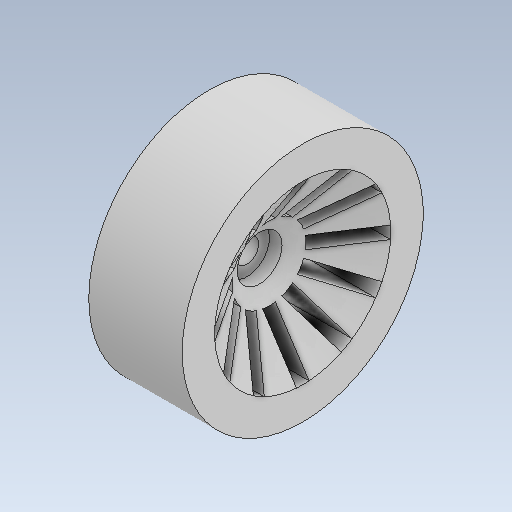
# Autodesk Inventor part: 04_Wheel
Saved by Autodesk Inventor 2021 (Build 250183000, 183)
## iProperties
Created: 2021-03-22
Part Number: 04_Wheel
Material: Generisch
Document SubType Name: Modeling
Designer: User
Density: 1 g/cm^3
Appearance: Vorgabe
Author: User
Autodesk Inventor part; units mm, degrees
ref_plane "YZ Plane" through (0, 0, 0) normal (1, 0, 0) x (0, 1, 0)
ref_plane "XZ Plane" through (0, 0, 0) normal (0, 1, 0) x (-1, 0, 0)
ref_plane "XY Plane" through (0, 0, 0) normal (0, 0, 1) x (1, 0, 0)
derived "00_Mastersketch.ipt"
sketch "05_wheelSketch" plane through (67, -17.95, 0) normal (0, 1, 0) x (-1, 0, 0)
  line L0 (-30, 33.5) -> (-4, 33.5) construction
  line L1 (-4, 33.5) -> (-4, -33.5) construction
  line L2 (-4, -33.5) -> (-30, -33.5) construction
  line L3 (-30, -33.5) -> (-30, 33.5) construction
  line L4 (-18, 16) -> (-30, 33.5) construction
  line L5 (-18, -16) -> (-18, 16) construction
  line L6 (-30, -33.5) -> (-18, -16) construction
  line L7 (-18, -6.25) -> (-4, -6.25) construction
  line L8 (-18, 6.25) -> (-4, 6.25) construction
  line L9 (-4, 0) -> (-30, 0)
  line L10 (-4, 33.5) -> (-30, 33.5)
  line L11 (-4, 33.5) -> (-4, 24.5)
  line L12 (-4, 24.5) -> (-30, 24.5)
  line L13 (-30, 24.5) -> (-30, 33.5)
  line L14 (-30, 24.5) -> (-18, 6.25)
  line L15 (-11, 24.5) -> (-11, 6.25)
  line L16 (-11, 6.25) -> (-18, 6.25)
  line L17 (-14.5, 6.25) -> (-14.5, 3.25)
  line L18 (-14.5, 3.25) -> (-11, 3.25)
  line L19 (-11, 3.25) -> (-11, 6.25)
  point P0 (67, 0)
  point P1 (-80.175, 24.1065)
  dimension "d1" = 9
  dimension "d10" = 3
  measures "d1" distance of L12.end L0.start
  measures "d10" distance between parallel lines of L18 L8
revolve "Umdrehung1" add sketch "05_wheelSketch" angle 360 about axis through (71, -17.95, 0) along (1, 0, 0)
sketch "Skizze2" plane through (97, -17.95, 0) normal (1, 0, 0) x (0, 0, -1)
  circle A0 centre (0, 0) radius 24.5 projected
  line L0 (-10.0995, -1.75) -> (-24.4374, -1.75)
  line L1 (-10.0995, 1.75) -> (-24.4374, 1.75)
  line L2 (0, 0) -> (-24.5, 0) construction
  circle A1 centre (0, 0) radius 10.25
  circle A2 centre (0, 0) radius 6.25 projected
  point P0 (0, 17.95)
  dimension "d3" = 3.5
  dimension "d14" = 4
  constraints: 6 end point, 5 point on circle, 2 coincident, 2 parallel, 1 centre point, 1 horizontal, 1 other
  measures "d3" distance between parallel lines of L0 L1
  measures "d14" radial gap between concentric circles of A1 A2
extrude "Extrusion1" cut sketch "Skizze2" against normal through all contours L1 A1 L0 A0 picked at (-14.9865, -0.1946)
pattern_circular "Runde Anordnung1" count 12 over 360 about axis through (84, -17.95, 0) along (-1, 0, 0) of "Extrusion1"
